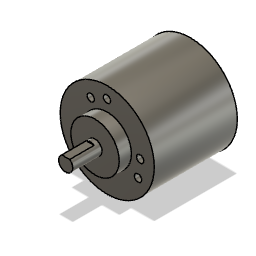
REMcontainer (Autodesk Fusion 360 archive; units mm, degrees)
design "RE"
Autodesk Fusion 360 part; units mm, degrees
cylinder "CylinderPrimitive1" add diameter 38.5 height 34 placed x (1, 0, 0) y (0, 1, 0) z (0, 0, 1) at (0, 0, 0)
cylinder "CylinderPrimitive2" add diameter 19.8 height 5 placed x (1, 0, 0) y (0, 1, 0) z (0, 0, 1) at (0, 0, 34)
cylinder "CylinderPrimitive3" add diameter 5.8 height 12 placed x (1, 0, 0) y (0, 1, 0) z (0, 0, 1) at (0, 0, 39)
sketch "Sketch4" plane through (0, 0, 34) normal (0, 0, 1) x (1, 0, 0)
  circle A0 centre (0, 0) radius 9.9
  circle A1 centre (0, 0) radius 19.25
  circle A2 centre (13.5, 0) radius 1.5
  line L0 (13.5, 0) -> (0, 0) construction
  line L1 (0, 0) -> (12.617, -7.1457) construction
  circle A3 centre (12.617, -7.1457) radius 1.5
  circle A4 centre (-6.75, 11.6913) radius 1.5
  circle A5 centre (-0.1202, 14.4995) radius 1.5
  circle A6 centre (-6.75, -11.6913) radius 1.5
  circle A7 centre (-12.4968, -7.3538) radius 1.5
  dimension "d7" = 3
  dimension "d8" = 13.5
  dimension "d9" = 14.5
  dimension "d10" = 7.2
  dimension "d12" = 360
  constraint coincident A2.centre L0.start
  constraint coincident A0.centre A1.centre
  constraint horizontal L0
  constraint coincident L1.end A3.centre
  constraint equal A2 A3
  measures "d7" diameter of A2
  measures "d8" distance of A0.centre A2.centre
  measures "d9" distance of A0.centre L1.end
  measures "d10" distance of A2.centre L1.end
extrude "Extrude1" cut sketch "Sketch4" against normal blind 5 contours A2 | A3 | A4 | A5 | A6 | A7
sketch "Sketch5" plane through (0, 0, 51) normal (0, 0, 1) x (1, 0, 0)
  circle A0 centre (0, 0) radius 2.9
  line L0 (-1.6279, 2.4) -> (1.6279, 2.4)
  dimension "d15" = 2.4
  constraint coincident A0 L0.start
  constraint coincident A0 L0.end
  constraint horizontal L0
  measures "d15" distance of A0.centre L0
extrude "Extrude2" cut sketch "Sketch5" against normal blind 10 contours A0 L0 picked at (0.1435, 2.556)
equation "d15 = ( 5.8 / 2 ) * 1 mm - 0.5 mm"
